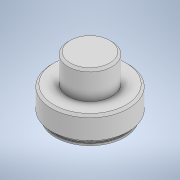
# Autodesk Inventor part: for_09G_-_axle_seal_installer
Saved by Autodesk Inventor 2021.2 (Build 252289000, 289)
## iProperties
Created: 2025-02-22
Part Number: for_09G_-_axle_seal_installer
Material: Generic
Document SubType Name: Modeling
Designer: Andrew
Density: 1 g/cm^3
Appearance: Default
Author: Andrew
Autodesk Inventor part; units mm, degrees
ref_plane "YZ Plane" through (0, 0, 0) normal (1, 0, 0) x (0, 1, 0)
ref_plane "XZ Plane" through (0, 0, 0) normal (0, 1, 0) x (-1, 0, 0)
ref_plane "XY Plane" through (0, 0, 0) normal (0, 0, 1) x (1, 0, 0)
sketch "Sketch1" plane through (0, 0, 0) normal (0, 0, 1) x (1, 0, 0)
  line L0 (31.65, 0) -> (35, 0)
  line L1 (35, 0) -> (35, 20.1)
  line L2 (35, 20.1) -> (12.65, 20.1)
  line L3 (12.65, 20.1) -> (12.65, 10.1)
  line L4 (12.65, 10.1) -> (31.65, 10.1)
  line L5 (31.65, 10.1) -> (31.65, 0)
  line L6 (22.5, 10) -> (31.5, 10)
  line L7 (31.5, 10) -> (31.5, 0)
  line L8 (31.5, 0) -> (22.5, 0)
  line L9 (22.5, 0) -> (22.5, 10)
  line L10 (12.5, 10.1) -> (12.5, 20.2)
  line L11 (12.5, 20.2) -> (19.939, 20.2)
  line L12 (19.939, 20.2) -> (19.939, 45.6)
  line L13 (19.939, 45.6) -> (0, 45.6)
  line L14 (7.65, 30.1) -> (7.65, 10.1)
  line L15 (7.65, 10.1) -> (12.5, 10.1)
  line L16 (0, 30) -> (7.5, 30)
  line L17 (7.5, 30) -> (7.5, 10)
  line L18 (7.5, 10) -> (15.4, 10)
  line L19 (15.4, 10) -> (15.4, -15)
  line L20 (15.4, -15) -> (0, -15)
  line L21 (0, -15) -> (0, 30)
  line L22 (22.5, -2.5) -> (31.5, -2.5)
  line L23 (31.5, -2.5) -> (31.5, -3.5)
  line L24 (31.5, -3.5) -> (22.5, -3.5)
  line L25 (22.5, -3.5) -> (22.5, -2.5)
  line L26 (22.5, -4.5) -> (31.5, -4.5)
  line L27 (31.5, -4.5) -> (31.5, -6.5)
  line L28 (31.5, -6.5) -> (22.5, -6.5)
  line L29 (22.5, -6.5) -> (22.5, -4.5)
  line L30 (22.5, -1) -> (31.5, -1)
  line L31 (31.5, -1) -> (31.5, -1.5)
  line L32 (31.5, -1.5) -> (22.5, -1.5)
  line L33 (22.5, -1.5) -> (22.5, -1)
  line L34 (0, 45.6) -> (0, 30.1)
  line L35 (0, 30.1) -> (7.65, 30.1)
  point P0 (0, 0)
  dimension "d0" = 35
  dimension "d1" = 19.939
  dimension "d2" = 12.5
  dimension "d3" = 7.5
  dimension "d5" = 22.5
  dimension "d7" = 31.5
  dimension "d8" = 0.1
  dimension "d9" = 0.15
  dimension "d10" = 10
  dimension "d11" = 0.15
  dimension "d12" = 0.1
  dimension "d13" = 10
  dimension "d14" = 0.15
  dimension "d15" = 0.1
  dimension "d16" = 25.4
  dimension "d17" = 20
  dimension "d19" = 15
  dimension "d20" = 15.4
  dimension "d21" = 1
  dimension "d22" = 2
  dimension "d23" = 0.5
  dimension "d24" = 1
  dimension "d25" = 1
  dimension "d26" = 1
  dimension "d27" = 0.1
  constraints: 72 end point, 21 perpendicular, 7 parallel, 7 point on line, 5 collinear, 5 horizontal, 2 vertical
  measures "d0" distance from line of point (0, 0) L1
  measures "d1" distance from line of point (0, 0) L12
  measures "d2" distance from line of point (0, 0) L10
  measures "d3" distance between parallel lines of L21 L17
  measures "d5" distance from line of L9 point (0, 0)
  measures "d7" distance from line of point (0, 0) L7
  measures "d8" distance between parallel lines of L6 L4
  measures "d9" distance between parallel lines of L5 L7
  measures "d10" distance of L8.end L6.start
  measures "d11" distance between parallel lines of L3 L10
  measures "d12" distance between parallel lines of L2 L11
  measures "d13" distance between parallel lines of L4 L2
  measures "d14" distance between parallel lines of L17 L14
  measures "d15" distance between parallel lines of L18 L15
  measures "d16" distance of L11.end L12.end
  measures "d17" distance between parallel lines of L18 L16
  measures "d19" distance from line of L20 point (0, 0)
  measures "d20" distance of L19.end L20.end
  measures "d21" distance of L24.end L22.start
  measures "d22" distance of L28.end L26.start
  measures "d23" distance of L32.end L30.start
  measures "d24" distance between parallel lines of L30 L8
  measures "d25" distance between parallel lines of L22 L32
  measures "d26" distance between parallel lines of L26 L24
  measures "d27" distance between parallel lines of L16 L35
revolve "Revolution1" add sketch "Sketch1" angle 360 about axis through (0, -15, 0) along (0, 1, 0)
chamfer "Chamfer1" distance 2 angle 45 3 edges at (-19.939, 45.6, 0) (-35, 20.1, 0) (-15.4, -15, 0)
equation "\"d8\" = y_tol"
equation "\"d9\" = x_tol"
equation "\"d11\" = x_tol"
equation "\"d12\" = y_tol"
equation "\"d14\" = x_tol"
equation "\"d15\" = y_tol"
equation "\"d27\" = y_tol"
equation "\"x_tol\" = 0.15"
equation "\"y_tol\" = 0.1"
body "Solid1"
